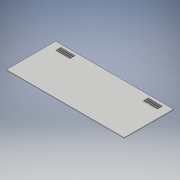
# Autodesk Inventor part: Peça21
Saved by Autodesk Inventor 2019 (Build 230136000, 136)
## iProperties
Created: 2020-03-11
Part Number: Peça21
Material: Aço, carbono
Document SubType Name: Modeling
Designer: caio.santos
Density: 7.85 g/cm^3
Appearance: Semipolido
Author: caio.santos
Autodesk Inventor part; units mm, degrees
ref_plane "YZ Plane" through (0, 0, 0) normal (1, 0, 0) x (0, 1, 0)
ref_plane "XZ Plane" through (0, 0, 0) normal (0, 1, 0) x (-1, 0, 0)
ref_plane "XY Plane" through (0, 0, 0) normal (0, 0, 1) x (1, 0, 0)
sketch "Esboço1" plane through (0, 0, 0) normal (0, 1, 0) x (-1, 0, 0)
  line L0 (215, 90) -> (-215, 90)
  line L1 (-215, 90) -> (-215, -90)
  line L2 (-215, -90) -> (215, -90)
  line L3 (215, -90) -> (215, 90)
  point P0 (0, 0)
  dimension "d3" = 180
  dimension "d5" = 215
  dimension "d6" = 430
  dimension "d7" = 90
  constraints: 8 end point, 2 perpendicular, 1 horizontal, 1 parallel
  measures "d3" distance of L0.end L1.end
  measures "d5" distance from line of L3 point (0, 0)
  measures "d6" distance of L1.end L2.end
  measures "d7" distance from line of point (0, 0) L0
extrude "Extrusão1" add sketch "Esboço1" along normal blind 2
sketch "Esboço2" plane through (0, 0, 0) normal (0, -1, 0) x (1, 0, 0)
  line L0 (215, -90) -> (-215, -90) projected
  line L1 (-215, -90) -> (-215, -89.25)
  line L2 (-215, -90) -> (-215, 90) projected
  line L3 (-215, -89.25) -> (215, -89.25)
  line L4 (215, 90) -> (215, -90) projected
  line L5 (215, -89.25) -> (215, -90)
  line L6 (215, -90) -> (-215, -90)
  point P0 (0, 0)
  dimension "d10" = 0.75
  dimension "d11" = 430
  constraints: 8 end point, 2 point on line, 1 collinear, 1 perpendicular
  measures "d10" distance of L0.end L1.end
  measures "d11" distance of L1.end L3.end
extrude "Extrusão2" add sketch "Esboço2" along normal blind 2
sketch "Esboço3" plane through (0, 2, 0) normal (0, 1, 0) x (1, 0, 0)
  line L0 (-215, 90) -> (215, 90) projected
  line L1 (-215, 80) -> (215, 80) construction
  line L2 (-215, 80) -> (-215, 60) construction
  line L3 (-215, 60) -> (215, 60) construction
  line L4 (215, 80) -> (215, 60) construction
  line L5 (-185, 60) -> (-182, 60) construction
  line L6 (-182, 60) -> (-182, 80) construction
  line L7 (-182, 80) -> (-185, 80) construction
  line L8 (-185, 80) -> (-185, 60) construction
  line L9 (-183.5, 60) -> (-183.5, 80) construction
  line L10 (-182, 61.5) -> (-182, 78.5)
  line L11 (-185, 78.5) -> (-185, 61.5)
  arc A0 (-185, 61.5) -> (-182, 61.5) centre (-183.5, 61.5) ccw
  arc A1 (-182, 78.5) -> (-185, 78.5) centre (-183.5, 78.5) ccw
  line L12 (-179, 78.5) -> (-179, 61.5)
  arc A2 (-176, 78.5) -> (-179, 78.5) centre (-177.5, 78.5) ccw
  line L13 (-176, 61.5) -> (-176, 78.5)
  arc A3 (-179, 61.5) -> (-176, 61.5) centre (-177.5, 61.5) ccw
  line L14 (-173, 78.5) -> (-173, 61.5)
  arc A4 (-170, 78.5) -> (-173, 78.5) centre (-171.5, 78.5) ccw
  line L15 (-170, 61.5) -> (-170, 78.5)
  arc A5 (-173, 61.5) -> (-170, 61.5) centre (-171.5, 61.5) ccw
  line L16 (-167, 78.5) -> (-167, 61.5)
  arc A6 (-164, 78.5) -> (-167, 78.5) centre (-165.5, 78.5) ccw
  line L17 (-164, 61.5) -> (-164, 78.5)
  arc A7 (-167, 61.5) -> (-164, 61.5) centre (-165.5, 61.5) ccw
  line L18 (-161, 78.5) -> (-161, 61.5)
  arc A8 (-158, 78.5) -> (-161, 78.5) centre (-159.5, 78.5) ccw
  line L19 (-158, 61.5) -> (-158, 78.5)
  arc A9 (-161, 61.5) -> (-158, 61.5) centre (-159.5, 61.5) ccw
  line L20 (-155, 78.5) -> (-155, 61.5)
  arc A10 (-152, 78.5) -> (-155, 78.5) centre (-153.5, 78.5) ccw
  line L21 (-152, 61.5) -> (-152, 78.5)
  arc A11 (-155, 61.5) -> (-152, 61.5) centre (-153.5, 61.5) ccw
  line L22 (-149, 78.5) -> (-149, 61.5)
  arc A12 (-146, 78.5) -> (-149, 78.5) centre (-147.5, 78.5) ccw
  line L23 (-146, 61.5) -> (-146, 78.5)
  arc A13 (-149, 61.5) -> (-146, 61.5) centre (-147.5, 61.5) ccw
  line L24 (-143, 78.5) -> (-143, 61.5)
  arc A14 (-140, 78.5) -> (-143, 78.5) centre (-141.5, 78.5) ccw
  line L25 (-140, 61.5) -> (-140, 78.5)
  arc A15 (-143, 61.5) -> (-140, 61.5) centre (-141.5, 61.5) ccw
  line L26 (-137, 78.5) -> (-137, 61.5)
  arc A16 (-134, 78.5) -> (-137, 78.5) centre (-135.5, 78.5) ccw
  line L27 (-134, 61.5) -> (-134, 78.5)
  arc A17 (-137, 61.5) -> (-134, 61.5) centre (-135.5, 61.5) ccw
  line L28 (185, 60) -> (182, 60) construction
  line L29 (182, 60) -> (182, 80) construction
  line L30 (182, 80) -> (185, 80) construction
  line L31 (185, 80) -> (185, 60) construction
  line L32 (183.5, 80) -> (183.5, 60) construction
  line L33 (182, 78.5) -> (182, 61.5)
  line L34 (185, 61.5) -> (185, 78.5)
  arc A18 (185, 78.5) -> (182, 78.5) centre (183.5, 78.5) ccw
  arc A19 (182, 61.5) -> (185, 61.5) centre (183.5, 61.5) ccw
  arc A20 (179, 78.5) -> (176, 78.5) centre (177.5, 78.5) ccw
  line L35 (179, 61.5) -> (179, 78.5)
  line L36 (176, 78.5) -> (176, 61.5)
  arc A21 (176, 61.5) -> (179, 61.5) centre (177.5, 61.5) ccw
  arc A22 (173, 78.5) -> (170, 78.5) centre (171.5, 78.5) ccw
  line L37 (173, 61.5) -> (173, 78.5)
  line L38 (170, 78.5) -> (170, 61.5)
  arc A23 (170, 61.5) -> (173, 61.5) centre (171.5, 61.5) ccw
  arc A24 (167, 78.5) -> (164, 78.5) centre (165.5, 78.5) ccw
  line L39 (167, 61.5) -> (167, 78.5)
  line L40 (164, 78.5) -> (164, 61.5)
  arc A25 (164, 61.5) -> (167, 61.5) centre (165.5, 61.5) ccw
  arc A26 (161, 78.5) -> (158, 78.5) centre (159.5, 78.5) ccw
  line L41 (161, 61.5) -> (161, 78.5)
  line L42 (158, 78.5) -> (158, 61.5)
  arc A27 (158, 61.5) -> (161, 61.5) centre (159.5, 61.5) ccw
  arc A28 (155, 78.5) -> (152, 78.5) centre (153.5, 78.5) ccw
  line L43 (155, 61.5) -> (155, 78.5)
  line L44 (152, 78.5) -> (152, 61.5)
  arc A29 (152, 61.5) -> (155, 61.5) centre (153.5, 61.5) ccw
  arc A30 (149, 78.5) -> (146, 78.5) centre (147.5, 78.5) ccw
  line L45 (149, 61.5) -> (149, 78.5)
  line L46 (146, 78.5) -> (146, 61.5)
  arc A31 (146, 61.5) -> (149, 61.5) centre (147.5, 61.5) ccw
  arc A32 (143, 78.5) -> (140, 78.5) centre (141.5, 78.5) ccw
  line L47 (143, 61.5) -> (143, 78.5)
  line L48 (140, 78.5) -> (140, 61.5)
  arc A33 (140, 61.5) -> (143, 61.5) centre (141.5, 61.5) ccw
  arc A34 (137, 78.5) -> (134, 78.5) centre (135.5, 78.5) ccw
  line L49 (137, 61.5) -> (137, 78.5)
  line L50 (134, 78.5) -> (134, 61.5)
  arc A35 (134, 61.5) -> (137, 61.5) centre (135.5, 61.5) ccw
  point P0 (0, 0)
  point P1 (-183.5, 70)
  point P2 (183.5, 70)
  dimension "d15" = 430
  dimension "d16" = 20
  dimension "d19" = 6
  dimension "d26" = 6
  dimension "d31" = 20
  dimension "d33" = 3
  dimension "d35" = 15
  dimension "d37" = 1.5
  dimension "d38" = 20
  dimension "d39" = 3
  dimension "d40" = 30
  dimension "d41" = 30
  dimension "d42" = 10
  dimension "d43" = 1.5
  constraints: 104 end point, 76 point on circle, 36 centre point, 8 tangent, 7 point on line, 6 midpoint, 6 parallel, 4 horizontal, 2 perpendicular, 160 other
  measures "d15" distance of L1.start L1.end
  measures "d16" distance of L1.start L2.end
  measures "d19" distance of L11.start L12.start
  measures "d26" distance of A18.centre A20.centre
  measures "d31" distance of L7.end L5.start
  measures "d33" distance between parallel lines of L12 L6
  measures "d35" distance between parallel lines of L15 L8
  measures "d37" radius of A18
  measures "d38" distance of L32.start L32.end
  measures "d39" distance between parallel lines of L35 L29
  measures "d40" distance between parallel lines of L4 L31
  measures "d41" distance between parallel lines of L2 L8
  measures "d42" distance from line of L0 L32.start
  measures "d43" radius of A2
extrude "Extrusão3" cut sketch "Esboço3" against normal blind 4
equation "\"d3\" = 2 * d7"
equation "\"d6\" = 2 * d5"
